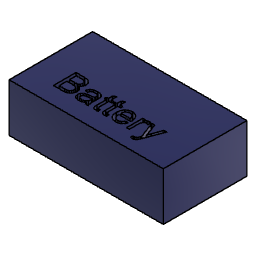
Battery 9V v2 (Autodesk Fusion 360 design; units mm, degrees)
Autodesk Fusion 360 part; units mm, degrees
sketch "Sketch1" plane through (0, 0, 0) normal (0, 0, 1) x (1, 0, 0)
  line L0 (0, 0) -> (48, 0)
  line L1 (48, 0) -> (48, 26)
  line L2 (48, 26) -> (0, 26)
  line L3 (0, 26) -> (0, 0)
  dimension "d1" = 48
  dimension "d2" = 26
  constraint horizontal L0
  constraint vertical L1
  constraint horizontal L2
  constraint vertical L3
  constraint coincident L0.start L3.end
  measures "d1" distance of L0.start L0.end
  measures "d2" distance of L0.start L2.end
extrude "Extrude1" add sketch "Sketch1" along normal blind 15
sketch "Text" plane through (0, 0, 15) normal (0, 0, 1) x (-1, 0, 0)
  line L0 (0, -26) -> (0, 0)
  line L1 (0, 0) -> (-48, 0)
  line L2 (-48, 0) -> (-48, -26)
  line L3 (-48, -26) -> (0, -26)
  line L4 (-8.4412, -5.8676) -> (-43.5652, -5.8676) construction
  line L5 (-43.5652, -5.8676) -> (-43.5652, -12.3721) construction
  line L6 (-43.5652, -12.3721) -> (-8.4412, -12.3721) construction
  line L7 (-8.4412, -12.3721) -> (-8.4412, -5.8676) construction
  dimension "d5" = 7
  text T0 "Battery" font "Arial" height 7 align left top in box 35.124 x 6.5045 at (-8.4412, -5.8676) x (-1, 0) y (0, -1) spacing 1
extrude "Extrude2" cut sketch "Text" against normal blind 2 text T0
